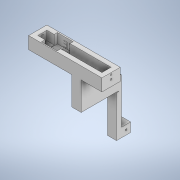
# Autodesk Inventor part: ArmAcrossPrint
Saved by Autodesk Inventor 2020 (Build 240168000, 168)
## iProperties
Created: 2020-01-21
Part Number: ArmAcrossPrint
Material: Generic
Document SubType Name: Modeling
Designer: tdmp4
Density: 1 g/cm^3
Appearance: Default
Author: tdmp4
Autodesk Inventor part; units mm, degrees
note: some values were not read from the file. Chosen so that the rebuilt part matches the saved one: direction of "Emboss1".
ref_plane "YZ Plane" through (0, 0, 0) normal (1, 0, 0) x (0, 1, 0)
ref_plane "XZ Plane" through (0, 0, 0) normal (0, 1, 0) x (-1, 0, 0)
ref_plane "XY Plane" through (0, 0, 0) normal (0, 0, 1) x (1, 0, 0)
sketch "Sketch1" plane through (0, 0, 0) normal (0, 1, 0) x (-1, 0, 0)
  line L0 (0, 0) -> (152.4, 0)
  line L1 (152.4, 0) -> (152.4, -38.1)
  line L2 (152.4, -38.1) -> (0, -38.1)
  line L3 (0, -38.1) -> (0, 0)
  dimension "d0" = 152.4
  dimension "d1" = 38.1
  constraints: 8 end point, 2 parallel, 1 horizontal, 1 perpendicular
  measures "d0" distance of L1.end L2.end
  measures "d1" distance of L2.end L0.start
extrude "Extrusion1" add sketch "Sketch1" along normal blind 25.4
sketch "Sketch3" plane through (0, 25.4, 0) normal (0, 1, 0) x (1, 0, 0)
  line L0 (-152.4, 0) -> (0, 0) projected
  line L1 (0, 0) -> (-9.525, 0)
  line L2 (-9.525, 0) -> (-9.525, 9.525)
  line L3 (-9.525, 9.525) -> (0, 9.525)
  line L4 (0, 9.525) -> (0, 0)
  line L5 (0, 38.1) -> (-152.4, 38.1) projected
  line L6 (-152.4, 38.1) -> (-142.875, 38.1)
  line L7 (-142.875, 38.1) -> (-142.875, 28.575)
  line L8 (-142.875, 28.575) -> (-152.4, 28.575)
  line L9 (-152.4, 28.575) -> (-152.4, 38.1)
  line L10 (-9.525, 9.525) -> (-142.875, 9.525)
  line L11 (-142.875, 9.525) -> (-142.875, 28.575)
  line L12 (-142.875, 28.575) -> (-9.525, 28.575)
  line L13 (-9.525, 28.575) -> (-9.525, 9.525)
  dimension "d4" = 9.525
  dimension "d5" = 9.525
  dimension "d6" = 9.525
  dimension "d7" = 9.525
  constraints: 24 end point, 6 parallel, 3 horizontal, 3 perpendicular
  measures "d4" distance of L2.end L3.end
  measures "d5" distance of L1.end L2.end
  measures "d6" distance of L7.end L8.end
  measures "d7" distance of L6.end L7.end
extrude "Extrusion2" cut sketch "Sketch3" against normal blind 19.05 contours L10 L11 L12 L13
sketch "Sketch4" plane through (0, 0, 0) normal (1, 0, 0) x (0, 0, -1)
  circle A0 centre (19.05, 21.5294) radius 1.7907
  circle A1 centre (19.05, 13.1683) radius 1.7907
  point P0 (0, 0)
  dimension "d24" = 3.5814
  dimension "d25" = 3.5814
  constraints: 2 centre point
  measures "d24" diameter of A0
  measures "d25" diameter of A1
extrude "Extrusion3" cut sketch "Sketch4" against normal blind 192.0875
sketch "Sketch5" plane through (0, 6.35, 0) normal (0, 1, 0) x (1, 0, 0)
  line L0 (0, 0) -> (0, 38.1) projected
  line L1 (0, 19.05) -> (-152.4, 19.05)
  line L2 (-152.4, 38.1) -> (-152.4, 0) projected
  circle A0 centre (-112.3138, 19.05) radius 9.779
  circle A1 centre (-122.0928, 19.05) radius 1.7907
  circle A2 centre (-102.5348, 19.05) radius 1.7907
  circle A3 centre (-112.3138, 29.2997) radius 1.7907
  circle A4 centre (-112.3138, 9.271) radius 1.7907
  dimension "d31" = 19.558
  dimension "d32" = 3.5814
  dimension "d33" = 3.5814
  dimension "d34" = 3.5814
  dimension "d35" = 3.5814
  constraints: 5 centre point, 3 point on circle, 3 point on line, 2 end point, 2 midpoint
  measures "d31" diameter of A0
  measures "d32" diameter of A1
  measures "d33" diameter of A2
  measures "d34" diameter of A3
  measures "d35" diameter of A4
extrude "Extrusion4" cut sketch "Sketch5" against normal blind 192.0875 contours A2 A0 L1 | L1 A0 A2 | A0 A2 L1 | L1 A2 A0 | A3 A0 | A0 A3 | A4 A0 | A0 A4 | A1 A0 L1 | L1 A0 A1 | A0 A1 L1 | L1 A1 A0
sketch "Sketch6" plane through (0, 25.4, 0) normal (0, 1, 0) x (1, 0, 0)
  line L0 (-95.0511, 1.8932) -> (-127.7029, 1.8932)
  line L1 (-127.7029, 1.8932) -> (-127.7029, 35.2854)
  line L2 (-127.7029, 35.2854) -> (-95.0511, 35.2854)
  line L3 (-95.0511, 35.2854) -> (-95.0511, 1.8932)
  point P0 (0, 0)
  constraints: 8 end point, 2 parallel, 1 horizontal, 1 perpendicular
extrude "Extrusion5" cut sketch "Sketch6" against normal blind 20.32
sketch "Sketch7" plane through (0, 0, 0) normal (0, -1, 0) x (1, 0, 0)
  line L0 (0, -38.1) -> (-152.4, -38.1) projected
  line L1 (-152.4, 0) -> (0, 0) projected
  line L2 (-55.8622, -38.1) -> (-62.2122, -38.1)
  line L3 (-62.2122, -38.1) -> (-62.2122, 0)
  line L4 (-62.2122, 0) -> (-55.8622, 0)
  line L5 (-55.8622, 0) -> (-55.8622, -38.1)
  dimension "d36" = 6.35
  constraints: 8 end point, 2 parallel, 2 point on line, 1 horizontal, 1 perpendicular
  measures "d36" distance of L3.end L4.end
extrude "Extrusion6" add sketch "Sketch7" along normal blind 58.42
sketch "Sketch8" plane through (0, 25.4, -38.1) normal (0, 0, -1) x (-1, 0, 0)
  line L0 (62.2122, -25.4) -> (62.2122, -83.82) projected
  line L1 (55.8622, -25.4) -> (55.8622, -83.82) projected
  line L2 (62.2122, -83.82) -> (55.8622, -83.82)
  line L3 (55.8622, -83.82) -> (55.8622, -58.1066)
  line L4 (55.8622, -58.1066) -> (62.2122, -58.1066)
  line L5 (62.2122, -58.1066) -> (62.2122, -83.82)
  point P0 (0, -25.4)
  constraints: 8 end point, 2 parallel, 1 horizontal, 1 perpendicular, 1 point on line
extrude "Extrusion7" add sketch "Sketch8" along normal blind 45.72
sketch "Sketch9" plane through (0, -58.42, 0) normal (0, -1, 0) x (1, 0, 0)
  line L0 (-62.2122, 0) -> (-62.2122, -83.82) projected
  line L1 (-55.8622, 0) -> (-55.8622, -83.82) projected
  line L2 (-62.2122, -83.82) -> (-55.8622, -83.82)
  line L3 (-55.8622, -83.82) -> (-55.8622, -77.4887)
  line L4 (-55.8622, -77.4887) -> (-62.2122, -77.4887)
  line L5 (-62.2122, -77.4887) -> (-62.2122, -83.82)
  point P0 (0, 0)
  constraints: 8 end point, 2 parallel, 1 horizontal, 1 perpendicular, 1 point on line
extrude "Extrusion8" add sketch "Sketch9" along normal blind 76.2
fillet "Fillet1" radius 1.5875 1 edges at (-59.0372, -58.42, -77.4887)
sketch "Sketch10" plane through (-55.8622, 0, 0) normal (1, 0, 0) x (0, 0, -1)
  line L0 (38.1, -32.7066) -> (83.82, -32.7066) projected
  line L1 (83.82, -32.7066) -> (38.1, 0)
  line L2 (38.1, 0) -> (38.1, -32.7066)
  line L3 (38.1, -32.7066) -> (83.82, -32.7066)
  point P0 (0, 0)
  constraints: 6 end point, 1 collinear, 1 perpendicular
extrude "Extrusion9" add sketch "Sketch10" against normal blind 6.35
sketch "Sketch11" plane through (-55.8622, -58.42, 0) normal (1, 0, 0) x (0, 0, -1)
  line L0 (83.82, 25.7134) -> (83.82, -76.2) projected
  line L1 (0, 0) -> (83.82, 0)
  line L2 (83.82, 0) -> (83.82, 25.7134)
  line L3 (83.82, 25.7134) -> (0, 25.7134)
  line L4 (0, 25.7134) -> (0, 0)
  line L5 (0, 58.42) -> (38.1, 58.42) projected
  line L6 (0, 58.42) -> (38.1, 58.42)
  line L7 (38.1, 58.42) -> (38.1, 25.7134)
  line L8 (38.1, 25.7134) -> (0, 25.7134)
  line L9 (0, 25.7134) -> (0, 58.42)
  line L10 (77.4887, -1.5875) -> (77.4887, -76.2) projected
  line L11 (83.82, 0) -> (77.4887, 0)
  line L12 (77.4887, 0) -> (77.4887, -76.2)
  line L13 (77.4887, -76.2) -> (83.82, -76.2)
  line L14 (83.82, -76.2) -> (83.82, 0)
  arc A0 (77.4887, -1.5875) -> (75.9012, 0) centre (75.9012, -1.5875) ccw projected
  arc A1 (77.4887, -1.5875) -> (75.9012, 0) centre (75.9012, -1.5875) ccw
  line L15 (38.1, 58.42) -> (83.82, 25.7134) projected
  line L16 (38.1, 58.42) -> (83.82, 25.7134)
  constraints: 26 end point, 7 equal length, 3 horizontal, 3 perpendicular, 2 point on circle, 1 centre point, 1 concentric, 1 point on line
extrude "Extrusion10" add sketch "Sketch11" along normal blind 12.7
sketch "Sketch14" plane through (0, -134.62, 0) normal (0, -1, 0) x (1, 0, 0)
  line L0 (-62.2122, -38.1) -> (-62.2122, -83.82) projected
  line L1 (-43.1622, -83.82) -> (-43.1622, -38.1) projected
  line L2 (-62.2122, -83.82) -> (-43.1622, -83.82)
  line L3 (-43.1622, -83.82) -> (-43.1622, -77.4782)
  line L4 (-43.1622, -77.4782) -> (-62.2122, -77.4782)
  line L5 (-62.2122, -77.4782) -> (-62.2122, -83.82)
  point P0 (0, 0)
  constraints: 8 end point, 2 parallel, 1 horizontal, 1 perpendicular, 1 point on line
extrude "Extrusion13" add sketch "Sketch14" along normal blind 11.3284
sketch "Sketch15" plane through (0, 25.4, -83.82) normal (0, 0, -1) x (-1, 0, 0)
  line L0 (43.1622, -171.3484) -> (62.2122, -171.3484) projected
  line L1 (62.2122, -171.3484) -> (43.1622, -171.3484)
  line L2 (43.1622, -171.3484) -> (43.1622, -152.2984)
  line L3 (43.1622, -152.2984) -> (62.2122, -152.2984)
  line L4 (62.2122, -152.2984) -> (62.2122, -171.3484)
  point P0 (0, -25.4)
  dimension "d57" = 19.05
  dimension "d58" = 19.05
  constraints: 8 end point, 2 parallel, 1 horizontal, 1 perpendicular
  measures "d57" distance of L1.end L2.end
  measures "d58" distance of L2.end L3.end
extrude "Extrusion14" add sketch "Sketch15" along normal blind 19.05
sketch "Sketch16" plane through (-43.1622, -58.42, 0) normal (1, 0, 0) x (0, 0, -1)
  line L0 (83.82, -68.4784) -> (102.87, -68.4784) projected
  line L1 (77.4782, -87.5284) -> (102.87, -87.5284) projected
  line L2 (83.82, -68.4784) -> (102.87, -87.5284)
  line L3 (102.87, -87.5284) -> (102.87, -68.4784) projected
  line L4 (102.87, -87.5284) -> (102.87, -68.4784)
  line L5 (102.87, -68.4784) -> (83.82, -87.5284)
  circle A0 centre (93.345, -78.0034) radius 1.7907
  point P0 (0, 58.42)
  dimension "d61" = 3.5814
  constraints: 6 end point, 1 centre point, 1 collinear, 1 midpoint
  measures "d61" diameter of A0
extrude "Extrusion15" cut sketch "Sketch16" against normal blind 39.6875 contours A0 L5 L2 | L2 L5 A0 | A0 L2 L5 | L2 A0 L5
sketch "Sketch17" plane through (-62.2122, -60.0075, -77.4887) normal (0, 0, 1) x (1, 0, 0)
  line L0 (0, -74.6125) -> (0, -85.9409) projected
  line L1 (19.05, 1.5875) -> (19.05, 0) projected
  line L2 (0, -85.9409) -> (19.05, -85.9409)
  line L3 (19.05, -85.9409) -> (19.05, 0)
  line L4 (19.05, 0) -> (0, 0)
  line L5 (0, 0) -> (0, -85.9409)
  point P0 (62.2122, 60.0075)
  constraints: 8 end point, 2 parallel, 1 horizontal, 1 perpendicular
extrude "Extrusion16" add sketch "Sketch17" along normal blind 3.9624
sketch "Sketch18" plane through (0, 25.4, -38.1) normal (0, 0, -1) x (-1, 0, 0)
  line L0 (41.8187, -6.5237) -> (122.4995, -6.5237)
  line L1 (122.4995, -6.5237) -> (122.4995, -19.7273)
  line L2 (122.4995, -19.7273) -> (41.8187, -19.7273)
  line L3 (41.8187, -19.7273) -> (41.8187, -6.5237)
  spline S0 degree 2 poles (51.828, -10.863) (51.828, -12.7618) (50.5685, -13.716) knots 0 0 0 1 1 1
  spline S1 degree 2 poles (50.5685, -13.716) (49.7193, -14.3553) (48.8796, -14.3553) knots 0 0 0 1 1 1
  line L4 (48.8796, -14.3553) -> (48.4407, -14.3553)
  line L5 (48.4407, -14.3553) -> (51.6658, -18.6681)
  spline S2 degree 2 poles (51.6658, -18.6681) (51.828, -18.9067) (51.828, -19.1357) knots 0 0 0 1 1 1
  spline S3 degree 2 poles (51.828, -19.1357) (51.828, -19.4219) (51.3795, -19.8704) (51.0837, -19.8704) knots 0 0 0 1 2 2 2
  spline S4 degree 2 poles (51.0837, -19.8704) (50.7211, -19.8704) (50.5685, -19.6414) knots 0 0 0 1 1 1
  line L6 (50.5685, -19.6414) -> (46.7804, -14.3553)
  line L7 (46.7804, -14.3553) -> (44.271, -14.3553)
  line L8 (44.271, -14.3553) -> (44.271, -19.1166)
  spline S5 degree 2 poles (44.271, -19.1166) (44.271, -19.8704) (43.5267, -19.8704) knots 0 0 0 1 1 1
  spline S6 degree 2 poles (43.5267, -19.8704) (42.792, -19.8704) (42.792, -19.1166) knots 0 0 0 1 1 1
  line L9 (42.792, -19.1166) -> (42.792, -7.2467)
  line L10 (42.792, -7.2467) -> (48.2021, -7.2467)
  spline S7 degree 2 poles (48.2021, -7.2467) (49.6716, -7.2467) (50.7116, -8.1914) knots 0 0 0 1 1 1
  spline S8 degree 2 poles (50.7116, -8.1914) (51.828, -9.2123) (51.828, -10.863) knots 0 0 0 1 1 1
  spline S9 degree 2 poles (50.3681, -10.863) (50.3681, -9.8707) (49.7193, -9.2696) knots 0 0 0 1 1 1
  spline S10 degree 2 poles (49.7193, -9.2696) (49.0991, -8.7162) (48.2021, -8.7162) knots 0 0 0 1 1 1
  line L11 (48.2021, -8.7162) -> (44.271, -8.7162)
  line L12 (44.271, -8.7162) -> (44.271, -12.8668)
  line L13 (44.271, -12.8668) -> (48.8796, -12.8668)
  spline S11 degree 2 poles (48.8796, -12.8668) (49.2803, -12.8668) (49.7288, -12.4851) knots 0 0 0 1 1 1
  spline S12 degree 2 poles (49.7288, -12.4851) (50.3681, -11.9413) (50.3681, -10.863) knots 0 0 0 1 1 1
  spline S13 degree 2 poles (63.7837, -18.8971) (63.8601, -19.0403) (63.8601, -19.2025) knots 0 0 0 1 1 1
  spline S14 degree 2 poles (63.8601, -19.2025) (63.8601, -19.9086) (63.0967, -19.9086) knots 0 0 0 1 1 1
  spline S15 degree 2 poles (63.0967, -19.9086) (62.6196, -19.9086) (62.4288, -19.4315) knots 0 0 0 1 1 1
  line L14 (62.4288, -19.4315) -> (61.6655, -17.5231)
  line L15 (61.6655, -17.5231) -> (55.5111, -17.5231)
  line L16 (55.5111, -17.5231) -> (54.7668, -19.4315)
  spline S16 degree 2 poles (54.7668, -19.4315) (54.5855, -19.9086) (54.0894, -19.9086) knots 0 0 0 1 1 1
  spline S17 degree 2 poles (54.0894, -19.9086) (53.3547, -19.9086) (53.3547, -19.1929) knots 0 0 0 1 1 1
  spline S18 degree 2 poles (53.3547, -19.1929) (53.3547, -19.0498) (53.3928, -18.9353) knots 0 0 0 1 1 1
  line L17 (53.3928, -18.9353) -> (57.6484, -7.6093)
  spline S19 degree 2 poles (57.6484, -7.6093) (57.8297, -7.1227) (58.4976, -7.1227) knots 0 0 0 1 1 1
  spline S20 degree 2 poles (58.4976, -7.1227) (59.1751, -7.1227) (59.3468, -7.5902) knots 0 0 0 1 1 1
  line L18 (59.3468, -7.5902) -> (63.7837, -18.8971)
  line L19 (61.1788, -16.0346) -> (58.4976, -9.1264)
  line L20 (58.4976, -9.1264) -> (55.9882, -16.0346)
  line L21 (55.9882, -16.0346) -> (61.1788, -16.0346)
  spline S21 degree 2 poles (75.6727, -19.1357) (75.6727, -19.8895) (74.9475, -19.8895) knots 0 0 0 1 1 1
  spline S22 degree 2 poles (74.9475, -19.8895) (74.2128, -19.8895) (74.2128, -19.1357) knots 0 0 0 1 1 1
  line L22 (74.2128, -19.1357) -> (74.2128, -9.5463)
  line L23 (74.2128, -9.5463) -> (71.3217, -14.1168)
  spline S23 degree 2 poles (71.3217, -14.1168) (70.9877, -14.6034) (70.5106, -14.6034) knots 0 0 0 1 1 1
  spline S24 degree 2 poles (70.5106, -14.6034) (70.0526, -14.6034) (69.8141, -14.2503) knots 0 0 0 1 1 1
  line L24 (69.8141, -14.2503) -> (66.8657, -9.5081)
  line L25 (66.8657, -9.5081) -> (66.8657, -19.1357)
  spline S25 degree 2 poles (66.8657, -19.1357) (66.8657, -19.8895) (66.1214, -19.8895) knots 0 0 0 1 1 1
  spline S26 degree 2 poles (66.1214, -19.8895) (65.3867, -19.8895) (65.3867, -19.1357) knots 0 0 0 1 1 1
  line L26 (65.3867, -19.1357) -> (65.3867, -8.0578)
  spline S27 degree 2 poles (65.3867, -8.0578) (65.3867, -7.2658) (66.1787, -7.2658) knots 0 0 0 1 1 1
  spline S28 degree 2 poles (66.1787, -7.2658) (66.7894, -7.2658) (67.1901, -7.8288) knots 0 0 0 1 1 1
  line L27 (67.1901, -7.8288) -> (70.5297, -12.7618)
  line L28 (70.5297, -12.7618) -> (73.9456, -7.7715)
  spline S29 degree 2 poles (73.9456, -7.7715) (74.3368, -7.1895) (74.8903, -7.1895) knots 0 0 0 1 1 1
  spline S30 degree 2 poles (74.8903, -7.1895) (75.6727, -7.1895) (75.6727, -8.0482) knots 0 0 0 1 1 1
  line L29 (75.6727, -8.0482) -> (75.6727, -19.1357)
  spline S31 degree 2 poles (81.245, -18.5727) (81.245, -19.0498) (80.5962, -19.67) (80.1477, -19.67) knots 0 0 0 1 2 2 2
  spline S32 degree 2 poles (80.1477, -19.67) (79.6707, -19.67) (79.0504, -19.0498) (79.0504, -18.5727) knots 0 0 0 1 2 2 2
  spline S33 degree 2 poles (79.0504, -18.5727) (79.0504, -18.1243) (79.6707, -17.485) (80.1477, -17.485) knots 0 0 0 1 2 2 2
  spline S34 degree 2 poles (80.1477, -17.485) (80.5962, -17.485) (81.245, -18.1338) (81.245, -18.5727) knots 0 0 0 1 2 2 2
  line L30 (92.5424, -19.7082) -> (84.8613, -19.7082)
  line L31 (84.8613, -19.7082) -> (84.8613, -7.2277)
  line L32 (84.8613, -7.2277) -> (92.5424, -7.2277)
  spline S35 degree 2 poles (92.5424, -7.2277) (93.2867, -7.2277) (93.2867, -7.9624) knots 0 0 0 1 1 1
  spline S36 degree 2 poles (93.2867, -7.9624) (93.2867, -8.7162) (92.5424, -8.7162) knots 0 0 0 1 1 1
  line L33 (92.5424, -8.7162) -> (86.3212, -8.7162)
  line L34 (86.3212, -8.7162) -> (86.3212, -12.1321)
  line L35 (86.3212, -12.1321) -> (92.1703, -12.1321)
  spline S37 degree 2 poles (92.1703, -12.1321) (92.9336, -12.1321) (92.9336, -12.8668) knots 0 0 0 1 1 1
  spline S38 degree 2 poles (92.9336, -12.8668) (92.9336, -13.6015) (92.1703, -13.6015) knots 0 0 0 1 1 1
  line L36 (92.1703, -13.6015) -> (86.3212, -13.6015)
  line L37 (86.3212, -13.6015) -> (86.3212, -18.2388)
  line L38 (86.3212, -18.2388) -> (92.5424, -18.2388)
  spline S39 degree 2 poles (92.5424, -18.2388) (93.2867, -18.2388) (93.2867, -18.9735) knots 0 0 0 1 1 1
  spline S40 degree 2 poles (93.2867, -18.9735) (93.2867, -19.7082) (92.5424, -19.7082) knots 0 0 0 1 1 1
  spline S41 degree 2 poles (104.5649, -18.7349) (104.6794, -18.9258) (104.6794, -19.1166) knots 0 0 0 1 1 1
  spline S42 degree 2 poles (104.6794, -19.1166) (104.6794, -19.4219) (104.2119, -19.8513) (103.9161, -19.8513) knots 0 0 0 1 2 2 2
  spline S43 degree 2 poles (103.9161, -19.8513) (103.5249, -19.8513) (103.4104, -19.6032) knots 0 0 0 1 1 1
  line L39 (103.4104, -19.6032) -> (99.9945, -14.1931)
  line L40 (99.9945, -14.1931) -> (96.6167, -19.5174)
  spline S44 degree 2 poles (96.6167, -19.5174) (96.3973, -19.8513) (96.0251, -19.8513) knots 0 0 0 1 1 1
  spline S45 degree 2 poles (96.0251, -19.8513) (95.7198, -19.8513) (95.2713, -19.4315) (95.2713, -19.1357) knots 0 0 0 1 2 2 2
  spline S46 degree 2 poles (95.2713, -19.1357) (95.2713, -18.9162) (95.3572, -18.7826) knots 0 0 0 1 1 1
  line L41 (95.3572, -18.7826) -> (99.1357, -12.9718)
  line L42 (99.1357, -12.9718) -> (96.216, -8.3059)
  spline S47 degree 2 poles (96.216, -8.3059) (96.1301, -8.1627) (96.1301, -7.9624) knots 0 0 0 1 1 1
  spline S48 degree 2 poles (96.1301, -7.9624) (96.1301, -7.6475) (96.6167, -7.2086) (96.903, -7.2086) knots 0 0 0 1 2 2 2
  spline S49 degree 2 poles (96.903, -7.2086) (97.2751, -7.2086) (97.5232, -7.6093) knots 0 0 0 1 1 1
  line L43 (97.5232, -7.6093) -> (99.9849, -11.7409)
  line L44 (99.9849, -11.7409) -> (102.4467, -7.5998)
  spline S50 degree 2 poles (102.4467, -7.5998) (102.6948, -7.2086) (103.0574, -7.2086) knots 0 0 0 1 1 1
  spline S51 degree 2 poles (103.0574, -7.2086) (103.3531, -7.2086) (103.8398, -7.657) (103.8398, -7.9624) knots 0 0 0 1 2 2 2
  spline S52 degree 2 poles (103.8398, -7.9624) (103.8398, -8.1532) (103.6776, -8.4204) knots 0 0 0 1 1 1
  line L45 (103.6776, -8.4204) -> (100.8341, -12.9718)
  line L46 (100.8341, -12.9718) -> (104.5649, -18.7349)
  line L47 (114.4979, -19.7082) -> (106.8168, -19.7082)
  line L48 (106.8168, -19.7082) -> (106.8168, -7.2277)
  line L49 (106.8168, -7.2277) -> (114.4979, -7.2277)
  spline S53 degree 2 poles (114.4979, -7.2277) (115.2421, -7.2277) (115.2421, -7.9624) knots 0 0 0 1 1 1
  spline S54 degree 2 poles (115.2421, -7.9624) (115.2421, -8.7162) (114.4979, -8.7162) knots 0 0 0 1 1 1
  line L50 (114.4979, -8.7162) -> (108.2767, -8.7162)
  line L51 (108.2767, -8.7162) -> (108.2767, -12.1321)
  line L52 (108.2767, -12.1321) -> (114.1257, -12.1321)
  spline S55 degree 2 poles (114.1257, -12.1321) (114.8891, -12.1321) (114.8891, -12.8668) knots 0 0 0 1 1 1
  spline S56 degree 2 poles (114.8891, -12.8668) (114.8891, -13.6015) (114.1257, -13.6015) knots 0 0 0 1 1 1
  line L53 (114.1257, -13.6015) -> (108.2767, -13.6015)
  line L54 (108.2767, -13.6015) -> (108.2767, -18.2388)
  line L55 (108.2767, -18.2388) -> (114.4979, -18.2388)
  spline S57 degree 2 poles (114.4979, -18.2388) (115.2421, -18.2388) (115.2421, -18.9735) knots 0 0 0 1 1 1
  spline S58 degree 2 poles (115.2421, -18.9735) (115.2421, -19.7082) (114.4979, -19.7082) knots 0 0 0 1 1 1
  point P0 (0, -25.4)
  constraints: 8 end point, 2 horizontal, 2 parallel, 1 perpendicular
emboss "Emboss1" sketch "Sketch18" operation cut depth 2.54 direction (0, 0, 1) contours S6 L9 L10 S7 S8 S0 S1 L4 L5 S2 S3 L2 S4 L6 L7 L8 S5 | L2 S5 S6 | S42 S43 L2 | L2 S43 L39 L40 S44 S45 S46 L41 L42 S47 S48 S49 L43 L44 S50 S51 S52 L45 L46 S41 S42 | L2 S3 S4 | S44 S45 L2 | S17 S18 L17 S19 S20 L18 S13 S14 L2 S15 L14 L15 L16 S16 | L2 S16 S17 | S21 S22 L2 | L2 S22 L22 L23 S23 S24 L24 L25 S25 S26 L26 S27 S28 L27 L28 S29 S30 L29 S21 | L2 S14 S15 | S25 S26 L2 | S31 S32 S33 S34 | L30 L31 L32 S35 S36 L33 L34 L35 S37 S38 L36 L37 L38 S39 S40 | L47 L48 L49 S53 S54 L50 L51 L52 S55 S56 L53 L54 L55 S57 S58
body "Solid1"
